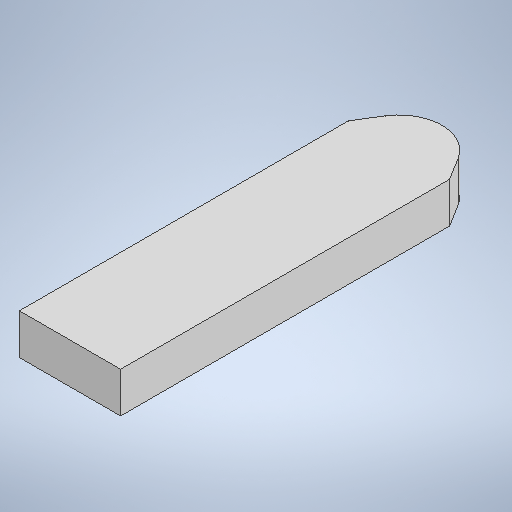
# Autodesk Inventor part: Servo_Shaft_select_V2
Saved by Autodesk Inventor 2025.3 (Build 293356000, 356)
## iProperties
Created: 2026-04-10
Part Number: Servo_Shaft_select_V2
Material: Generic
Document SubType Name: Modeling
Designer: kamal
Density: 1 g/cm^3
Appearance: Default
Mass: 5.65431 g
Surface Area: 27.7969 cm^2
Volume: 5.65431 cm^3
Author: kamal
## iProperties of the stored document Servo_Shaft_select_V2_3DPrint.ipt
Created: 2026-04-22
Part Number: Servo_Shaft_select_V2_3DPrint
Material: Generic
Document SubType Name: Modeling
Designer: kamal
Density: 1 g/cm^3
Appearance: Default
Author: kamal
Autodesk Inventor part; units mm, degrees
ref_plane "YZ Plane" through (0, 0, 0) normal (1, 0, 0) x (0, 1, 0)
ref_plane "XZ Plane" through (0, 0, 0) normal (0, 1, 0) x (-1, 0, 0)
ref_plane "XY Plane" through (0, 0, 0) normal (0, 0, 1) x (1, 0, 0)
sketch "Sketch1" plane through (0, 0, 0) normal (0, 1, 0) x (-1, 0, 0)
  arc A0 (-2.75, 2.165064) -> (2.75, 2.165064) centre (0, 0) ccw
  line L0 (-1.9, 14.1) -> (-2.75, 2.165064)
  line L1 (1.898718, 14.098684) -> (2.75, 2.165064)
  arc A1 (1.898718, 14.098684) -> (-1.9, 14.1) centre (-0.000658, 14.05) ccw
  circle A2 centre (0, 0) radius 0.5
  line L2 (0, 0) -> (0, -10) construction
  line L3 (0, 30) -> (0, 0) construction
  arc A3 (-7.653502, 3.697825) -> (7.653343, 3.698154) centre (0, 0) ccw
  line L4 (7.653343, 3.698154) -> (6.891627, 14.376202)
  arc A4 (6.891627, 14.376202) -> (-6.892842, 14.378331) centre (-0.000658, 14.05) ccw
  line L5 (-6.892842, 14.378331) -> (-7.653502, 3.697825)
  line L6 (10, 0) -> (-10, 0)
  line L7 (-10, 0) -> (-10, 30)
  line L8 (-10, 30) -> (10, 30)
  line L9 (10, 30) -> (10, 0)
  point P0 (-8.5, 0)
  point P1 (8.5, 0)
  dimension "d0" = 1
  dimension "d9" = 1.9
  dimension "d11" = 3.5
  dimension "d34" = 10
  dimension "d42" = 5
  dimension "d43" = 20
  dimension "d44" = 30
  constraints: 20 end point, 8 point on circle, 5 centre point, 2 perpendicular, 2 vertical, 1 coincident, 1 collinear, 1 concentric, 1 horizontal, 1 midpoint, 3 other
  measures "d0" diameter of A2
  measures "d9" radius of A1
  measures "d11" radius of A0
  measures "d34" distance of L2.start L2.end
  measures "d42" distance between parallel lines of L0 L5
  measures "d43" distance of L6.start L6.end
  measures "d44" distance of L6.end L7.end
sketch "Sketch1 outline for Extrusion6" plane through (0, 0, 0) normal (0, 1, 0) x (-1, 0, 0)
  arc A0 (-8.5, 0) -> (8.5, 0) centre (0, 0) ccw
  line L0 (-10, 0) -> (-8.5, 0)
  line L1 (8.5, 0) -> (10, 0)
  line L2 (-10, 30) -> (-10, 0)
  line L3 (10, 0) -> (10, 30)
  line L4 (10, 30) -> (-10, 30)
  arc A1 (2.75, 2.165064) -> (-2.75, 2.165064) centre (0, 0) cw
  line L5 (1.898718, 14.098684) -> (2.75, 2.165064)
  arc A2 (-1.9, 14.1) -> (1.898718, 14.098684) centre (-0.000658, 14.05) cw
  line L6 (-2.75, 2.165064) -> (-1.9, 14.1)
extrude "Extrusion6" add sketch "Sketch1 outline for Extrusion6" along normal blind 8
sketch "Sketch7" plane through (0, 0, 0) normal (0, -1, 0) x (1, 0, 0)
  arc A0 (-8.5, 0) -> (8.5, 0) centre (0, 0) ccw
  line L0 (10, 30) -> (10, 0)
  line L1 (-10, 0) -> (-10, 30)
  line L2 (-10, 0) -> (-10, 30)
  line L3 (-10, 0) -> (-7.225, -4.477653)
  line L4 (10, 0) -> (7.225, -4.477653)
  line L5 (8.5, 0) -> (10, 0)
  line L6 (-8.5, 0) -> (-10, 0)
  line L7 (-8.5, 0) -> (-10, 0)
  constraints: 8 end point, 3 point on circle, 2 collinear, 2 tangent
sketch "Sketch7 outline for Extrusion7" plane through (0, 0, 0) normal (0, -1, 0) x (1, 0, 0)
  line L0 (-8.5, 0) -> (-10, 0)
  arc A0 (-7.225, -4.477653) -> (-8.5, 0) centre (0, 0) cw
  line L1 (-10, 0) -> (-7.225, -4.477653)
  line L2 (10, 0) -> (8.5, 0)
  line L3 (7.225, -4.477653) -> (10, 0)
  arc A1 (8.5, 0) -> (7.225, -4.477653) centre (0, 0) cw
extrude "Extrusion7" add sketch "Sketch7 outline for Extrusion7" against normal blind 8
sketch "Sketch8" plane through (0, 0, 0) normal (0, -1, 0) x (1, 0, 0)
  line L0 (-10, 0) -> (-7.225, -4.477653)
  arc A0 (-7.225, -4.477653) -> (7.225, -4.477653) centre (0, 0) ccw
  line L1 (7.225, -4.477653) -> (10, 0)
  line L2 (10, 30) -> (10, 0)
  line L3 (-10, 30) -> (10, 30)
  line L4 (-10, 0) -> (-10, 30)
  arc A1 (-2.75, 2.165064) -> (2.75, 2.165064) centre (0, 0) ccw
  line L5 (-1.898718, 14.098684) -> (-2.75, 2.165064)
  arc A2 (1.9, 14.1) -> (-1.898718, 14.098684) centre (0.000658, 14.05) ccw
  line L6 (2.75, 2.165064) -> (1.9, 14.1)
  circle A3 centre (0, 20) radius 10
  line L7 (10, 30) -> (10, 1.423737)
  line L8 (-10, 30) -> (10, 30)
  point P0 (-10, 20)
  point P1 (0, 30)
  point P2 (10, 20)
  point P3 (2.174951, 10.239386)
  point P4 (-2.174035, 10.239182)
  dimension "d50" = 20
  constraints: 2 tangent, 1 centre point
  measures "d50" diameter of A3
sketch "Sketch8 outline for Extrusion8" plane through (0, 0, 0) normal (0, -1, 0) x (1, 0, 0)
  arc A0 (-10, 20) -> (0, 30) centre (0, 20) cw
  line L0 (-10, 30) -> (-10, 20)
  line L1 (0, 30) -> (-10, 30)
  arc A1 (0, 30) -> (10, 20) centre (0, 20) cw
  line L2 (10, 30) -> (0, 30)
  line L3 (10, 20) -> (10, 30)
extrude "Extrusion8" cut sketch "Sketch8 outline for Extrusion8" against normal through all
sketch "Sketch9" plane through (0, 8, 0) normal (0, 1, 0) x (1, 0, 0)
  arc A0 (-10, -20) -> (10, -20) centre (0, -20) ccw
  line L0 (-10, 0) -> (-10, -20)
  arc A1 (-9.25, 1.210176) -> (-10, -1.423737) centre (-5, -1.423737) ccw
  line L1 (-7.225, 4.477653) -> (-10, 0)
  arc A2 (7.225, 4.477653) -> (-7.225, 4.477653) centre (0, 0) ccw
  line L2 (10, 0) -> (7.225, 4.477653)
  arc A3 (10, -1.423737) -> (9.25, 1.210176) centre (5, -1.423737) ccw
  line L3 (10, -20) -> (10, 0)
sketch "Sketch9 outline for Extrusion9" plane through (0, 8, 0) normal (0, 1, 0) x (1, 0, 0)
  arc A0 (-10, -20) -> (10, -20) centre (0, -20) ccw
  line L0 (-10, -1.423737) -> (-10, -20)
  arc A1 (-9.25, 1.210176) -> (-10, -1.423737) centre (-5, -1.423737) ccw
  line L1 (-7.225, 4.477653) -> (-9.25, 1.210176)
  arc A2 (7.225, 4.477653) -> (-7.225, 4.477653) centre (0, 0) ccw
  line L2 (9.25, 1.210176) -> (7.225, 4.477653)
  arc A3 (10, -1.423737) -> (9.25, 1.210176) centre (5, -1.423737) ccw
  line L3 (10, -20) -> (10, -1.423737)
extrude "Extrusion9" add sketch "Sketch9 outline for Extrusion9" against normal blind 5
sketch "Sketch10" plane through (0, 0, 0) normal (0, -1, 0) x (1, 0, 0)
  line L0 (10, 20) -> (10, 0) projected
  line L1 (0, 0) -> (10, 0)
  line L2 (10, 0) -> (10, 65)
  line L3 (10, 65) -> (0, 65)
  line L4 (0, 65) -> (0, 0) construction
  line L5 (-10, 0) -> (-10, 20) projected
  line L6 (0, 0) -> (-10, 0)
  line L7 (-10, 0) -> (-10, 65)
  line L8 (-10, 65) -> (0, 65)
  dimension "d55" = 65
  constraints: 14 end point, 3 perpendicular, 2 horizontal, 2 parallel
  measures "d55" distance of L2.end L0.end
sketch "Sketch10 outline for Extrusion10" plane through (0, 0, 0) normal (0, -1, 0) x (1, 0, 0)
  line L0 (-10, 0) -> (0, 0)
  line L1 (-10, 20) -> (-10, 0)
  line L2 (-10, 65) -> (-10, 20)
  line L3 (0, 65) -> (-10, 65)
  line L4 (10, 65) -> (0, 65)
  line L5 (10, 20) -> (10, 65)
  line L6 (10, 0) -> (10, 20)
  line L7 (0, 0) -> (10, 0)
extrude "Extrusion10" add sketch "Sketch10 outline for Extrusion10" against normal blind 8
sketch "Sketch8 outline for Extrusion11" plane through (0, 0, 0) normal (0, -1, 0) x (1, 0, 0)
  arc A0 (-2.75, 2.165064) -> (2.75, 2.165064) centre (0, 0) ccw
  line L0 (-2.174035, 10.239182) -> (-2.75, 2.165064)
  arc A1 (2.174951, 10.239386) -> (-2.174035, 10.239182) centre (0, 20) cw
  line L1 (2.75, 2.165064) -> (2.174951, 10.239386)
extrude "Extrusion11" cut sketch "Sketch8 outline for Extrusion11" against normal blind 3
sketch "Sketch8 outline for Extrusion12" plane through (0, 0, 0) normal (0, -1, 0) x (1, 0, 0)
  arc A0 (1.9, 14.1) -> (-1.898718, 14.098684) centre (0.000658, 14.05) ccw
  line L0 (2.174951, 10.239386) -> (1.9, 14.1)
  arc A1 (-2.174035, 10.239182) -> (2.174951, 10.239386) centre (0, 20) ccw
  line L1 (-1.898718, 14.098684) -> (-2.174035, 10.239182)
extrude "Extrusion12" cut sketch "Sketch8 outline for Extrusion12" against normal blind 3
body "Solid2"
